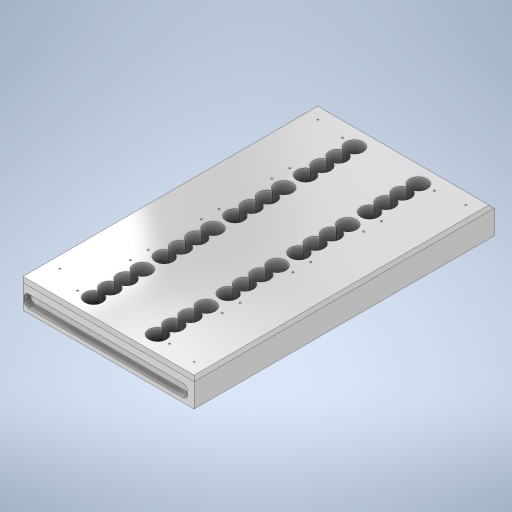
# Autodesk Inventor part: Assembly Plate
Saved by Autodesk Inventor 2023 (Build 270158000, 158)
## iProperties
Created: 2022-03-23
Part Number: Assembly Plate
Material: Generic
Document SubType Name: Modeling
Designer: Caleb
Density: 1 g/cm^3
Appearance: Aluminum - Dark
Author: Caleb
Autodesk Inventor part; units mm, degrees
ref_plane "YZ Plane" through (0, 0, 0) normal (1, 0, 0) x (0, 1, 0)
ref_plane "XZ Plane" through (0, 0, 0) normal (0, 1, 0) x (-1, 0, 0)
ref_plane "XY Plane" through (0, 0, 0) normal (0, 0, 1) x (1, 0, 0)
sketch "Sketch1" plane through (0, 0, 0) normal (0, 1, 0) x (-1, 0, 0)
  line L0 (-63.5, -107.95) -> (63.5, -107.95)
  line L1 (63.5, -107.95) -> (63.5, 107.95)
  line L2 (63.5, 107.95) -> (-63.5, 107.95)
  line L3 (-63.5, 107.95) -> (-63.5, -107.95)
  line L4 (-63.5, -107.95) -> (63.5, 107.95) construction
  line L5 (63.5, -107.95) -> (-63.5, 107.95) construction
  point P0 (0, 0)
  dimension "d0" = 127
  dimension "d1" = 215.9
  constraints: 12 end point, 2 midpoint, 2 parallel, 1 horizontal, 1 perpendicular
  measures "d0" distance of L2.end L1.end
  measures "d1" distance of L1.end L0.end
extrude "Extrusion1" add sketch "Sketch1" along normal blind 19.05
sketch "Sketch5" plane through (0, 19.05, 0) normal (0, 1, 0) x (1, 0, 0)
  line L0 (-63.5, -107.95) -> (63.5, -107.95) projected
  line L1 (63.5, 107.95) -> (-63.5, 107.95) projected
  line L2 (-63.5, 107.95) -> (-63.5, -107.95) projected
  line L3 (63.5, -107.95) -> (63.5, 107.95) projected
  point P0 (0, 0)
  point P1 (-53.15, -87.9)
  point P2 (-53.15, 97.6)
  point P3 (53.15, 97.6)
  point P4 (53.15, -97.6)
  dimension "d31" = 20.05
  dimension "d32" = 10.35
  dimension "d33" = 10.35
  dimension "d34" = 10.35
  dimension "d35" = 10.35
  dimension "d36" = 10.35
  dimension "d37" = 10.35
  dimension "d38" = 10.35
  measures "d31" distance from line of L0 point (-53.15, -87.9)
  measures "d32" distance from line of L0 point (53.15, -97.6)
  measures "d33" distance from line of L1 point (53.15, 97.6)
  measures "d34" distance from line of L1 point (-53.15, 97.6)
  measures "d35" distance from line of L2 point (-53.15, 97.6)
  measures "d36" distance from line of L3 point (53.15, 97.6)
  measures "d37" distance from line of L3 point (53.15, -97.6)
  measures "d38" distance from line of L2 point (-53.15, -87.9)
hole "Hole3" at (-53.15, 19.05, 87.9) at (-53.15, 19.05, -97.6) at (53.15, 19.05, -97.6) at (53.15, 19.05, 97.6) direction (0, -1, 0) diameter 1.0211 end through all thread size "00-96 NS" class "2B" standard "ANSI Unified Screw Threads"
sketch "Sketch6" plane through (0, 19.05, 0) normal (0, 1, 0) x (1, 0, 0)
  line L0 (-63.5, -107.95) -> (63.5, -107.95) projected
  line L1 (-63.5, 107.95) -> (-63.5, -107.95) projected
  point P0 (0, 0)
  point P1 (-25.75, -94.25)
  point P2 (-25.75, -58.15)
  point P3 (25.75, -58.15)
  point P4 (25.75, -94.25)
  point P5 (25.75, -43.45)
  point P6 (25.75, -7.35)
  point P7 (-25.75, -7.35)
  point P8 (-25.75, -43.45)
  point P9 (25.75, 7.35)
  point P10 (25.75, 43.45)
  point P11 (-25.75, 43.45)
  point P12 (-25.75, 7.35)
  point P13 (25.75, 58.15)
  point P14 (25.75, 94.25)
  point P15 (-25.75, 94.25)
  point P16 (-25.75, 58.15)
  dimension "d46" = 36.1
  dimension "d47" = 51.5
  dimension "d48" = 13.7
  dimension "d49" = 37.75
  dimension "d52" = 50.8
  constraints: 2 horizontal alignment, 2 vertical alignment, 1 vertical, 12 other
  measures "d46" distance of point (-25.75, -58.15) point (-25.75, -94.25)
  measures "d47" distance of point (25.75, -94.25) point (-25.75, -94.25)
  measures "d48" distance from line of L0 point (-25.75, -94.25)
  measures "d49" distance from line of L1 point (-25.75, -94.25)
  measures "d52" distance of point (25.75, -94.25) point (25.75, -43.45)
hole "Hole4" [suppressed]
sketch "Sketch8" plane through (63.5, 0, -107.95) normal (0, 0, -1) x (-1, 0, 0)
  line L0 (119.0625, 3.175) -> (7.9375, 3.175)
  line L1 (4.7625, 6.35) -> (4.7625, 8.89)
  line L2 (7.9375, 12.065) -> (119.0625, 12.065)
  line L3 (122.2375, 8.89) -> (122.2375, 6.35)
  line L4 (122.2375, 3.175) -> (4.7625, 12.065) construction
  line L5 (4.7625, 3.175) -> (122.2375, 12.065) construction
  line L6 (0, 0) -> (0, 19.05) projected
  line L7 (127, 0) -> (127, 19.05) projected
  line L8 (0, 0) -> (127, 0) projected
  arc A0 (7.9375, 12.065) -> (4.7625, 8.89) centre (7.9375, 8.89) ccw
  arc A1 (4.7625, 6.35) -> (7.9375, 3.175) centre (7.9375, 6.35) ccw
  arc A2 (119.0625, 3.175) -> (122.2375, 6.35) centre (119.0625, 6.35) ccw
  arc A3 (122.2375, 8.89) -> (119.0625, 12.065) centre (119.0625, 8.89) ccw
  point P0 (63.5, 0)
  point P1 (63.5, 7.62)
  point P2 (0, 15.875)
  point P3 (127, 15.875)
  dimension "d77" = 8.89
  dimension "d78" = 4.7625
  dimension "d79" = 4.7625
  dimension "d80" = 3.175
  dimension "d83" = 3.175
  constraints: 12 end point, 8 point on circle, 8 point on line, 8 tangent, 4 centre point, 3 equal radius, 2 midpoint, 2 parallel, 1 horizontal, 1 perpendicular
  measures "d77" distance of L5.start L4.end
  measures "d78" distance between parallel lines of L6 L1
  measures "d79" distance between parallel lines of L7 L3
  measures "d80" distance between parallel lines of L8 L0
  measures "d83" radius of A0
extrude "Extrusion4" cut sketch "Sketch8" against normal blind 4.7625
sketch "Sketch9" plane through (63.5, 0, 107.95) normal (0, 0, 1) x (1, 0, 0)
  line L0 (-7.9375, 3.175) -> (-119.0625, 3.175)
  line L1 (-122.2375, 6.35) -> (-122.2375, 8.89)
  line L2 (-119.0625, 12.065) -> (-7.9375, 12.065)
  line L3 (-4.7625, 8.89) -> (-4.7625, 6.35)
  line L4 (-4.7625, 3.175) -> (-122.2375, 12.065) construction
  line L5 (-122.2375, 3.175) -> (-4.7625, 12.065) construction
  arc A0 (-119.0625, 12.065) -> (-122.2375, 8.89) centre (-119.0625, 8.89) ccw
  arc A1 (-122.2375, 6.35) -> (-119.0625, 3.175) centre (-119.0625, 6.35) ccw
  arc A2 (-7.9375, 3.175) -> (-4.7625, 6.35) centre (-7.9375, 6.35) ccw
  arc A3 (-4.7625, 8.89) -> (-7.9375, 12.065) centre (-7.9375, 8.89) ccw
  line L6 (-127, 0) -> (0, 0) projected
  line L7 (-127, 0) -> (-127, 19.05) projected
  line L8 (0, 0) -> (0, 19.05) projected
  point P0 (63.5, 0)
  point P1 (-63.5, 7.62)
  point P2 (-123.825, 0)
  dimension "d84" = 8.89
  dimension "d88" = 3.175
  dimension "d89" = 3.175
  dimension "d93" = 4.7625
  dimension "d94" = 4.7625
  constraints: 12 end point, 8 point on circle, 8 point on line, 8 tangent, 4 centre point, 3 equal radius, 2 midpoint, 2 parallel, 1 horizontal, 1 perpendicular
  measures "d84" distance of L5.start L4.end
  measures "d88" radius of A0
  measures "d89" distance between parallel lines of L6 L0
  measures "d93" distance between parallel lines of L7 L1
  measures "d94" distance between parallel lines of L8 L3
extrude "Extrusion5" cut sketch "Sketch9" against normal blind 4.7625
sketch "Sketch10" plane through (0, 19.05, 0) normal (0, 1, 0) x (1, 0, 0)
  line L0 (63.5, -107.95) -> (63.5, 107.95) projected
  line L1 (-63.5, -107.95) -> (63.5, -107.95) projected
  line L2 (-63.5, 107.95) -> (-63.5, -107.95) projected
  line L3 (13.3831, -76.2) -> (-9.5437, -76.2) construction
  line L4 (0, -87.2187) -> (0, -59.9039) construction
  line L5 (13.3831, -25.4) -> (-9.5437, -25.4) construction
  line L6 (0, -36.4187) -> (0, -9.1039) construction
  line L7 (13.3831, 25.4) -> (-9.5437, 25.4) construction
  line L8 (0, 14.3813) -> (0, 41.6961) construction
  line L9 (13.3831, 76.2) -> (-9.5437, 76.2) construction
  line L10 (0, 65.1813) -> (0, 92.4961) construction
  point P0 (23, -93.7)
  point P1 (23, -82.0333)
  point P2 (-23, -93.7)
  point P3 (-23, -82.0333)
  point P4 (23, -70.3667)
  point P5 (-23, -70.3667)
  point P6 (23, -58.7)
  point P7 (-23, -58.7)
  point P8 (0, -76.2)
  point P9 (33, -95.2)
  point P10 (33, -57.2)
  point P11 (-33, -95.2)
  point P12 (-33, -57.2)
  point P13 (0, -25.4)
  point P14 (-33, -6.4)
  point P15 (-33, -44.4)
  point P16 (33, -6.4)
  point P17 (33, -44.4)
  point P18 (-23, -7.9)
  point P19 (23, -7.9)
  point P20 (-23, -19.5667)
  point P21 (23, -19.5667)
  point P22 (-23, -31.2333)
  point P23 (-23, -42.9)
  point P24 (23, -31.2333)
  point P25 (23, -42.9)
  point P26 (0, 25.4)
  point P27 (-33, 44.4)
  point P28 (-33, 6.4)
  point P29 (33, 44.4)
  point P30 (33, 6.4)
  point P31 (-23, 42.9)
  point P32 (23, 42.9)
  point P33 (-23, 31.2333)
  point P34 (23, 31.2333)
  point P35 (-23, 19.5667)
  point P36 (-23, 7.9)
  point P37 (23, 19.5667)
  point P38 (23, 7.9)
  point P39 (0, 76.2)
  point P40 (-33, 95.2)
  point P41 (-33, 57.2)
  point P42 (33, 95.2)
  point P43 (33, 57.2)
  point P44 (-23, 93.7)
  point P45 (23, 93.7)
  point P46 (-23, 82.0333)
  point P47 (23, 82.0333)
  point P48 (-23, 70.3667)
  point P49 (-23, 58.7)
  point P50 (23, 70.3667)
  point P51 (23, 58.7)
  dimension "d96" = 14.25
  dimension "d97" = 11.6667
  dimension "d127" = 11.6667
  dimension "d128" = 11.6667
  dimension "d129" = 46
  dimension "d130" = 35
  dimension "d131" = 17.5
  dimension "d132" = 23
  dimension "d133" = 33
  dimension "d134" = 19
  dimension "d135" = 38
  dimension "d136" = 33
  dimension "d146" = 50.8
  dimension "d154" = 63.5
  dimension "d155" = 127
  constraints: 16 end point, 8 point on line, 8 vertical alignment, 6 horizontal alignment, 2 perpendicular, 2 vertical, 1 horizontal, 57 other
  measures "d96" distance from line of point (23, -93.7) L1
  measures "d97" distance of point (23, -93.7) point (23, -82.033)
  measures "d127" distance of point (23, -82.033) point (23, -70.367)
  measures "d128" distance of point (23, -70.367) point (23, -58.7)
  measures "d129" distance of point (23, -93.7) point (-23, -93.7)
  measures "d130" distance of point (-23, -93.7) point (-23, -58.7)
  measures "d131" distance from line of point (-23, -58.7) L3
  measures "d132" distance from line of point (-23, -93.7) L4
  measures "d133" horizontal distance of point (33, -95.2) point (0, -76.2)
  measures "d134" vertical distance of point (33, -95.2) point (0, -76.2)
  measures "d135" distance of point (33, -57.2) point (33, -95.2)
  measures "d136" horizontal distance of point (-33, -95.2) point (0, -76.2)
  measures "d146" distance of L3.start L5.start
  measures "d154" distance from line of L0 point (0, -76.2)
  measures "d155" distance of L1.start L0.start
hole "Hole5" at (23, 19.05, 93.7) at (23, 19.05, 82.0333) at (-23, 19.05, 93.7) at (-23, 19.05, 82.0333) at (23, 19.05, 70.3667) at (23, 19.05, 58.7) at (-23, 19.05, 58.7) at (-23, 19.05, 70.3667) at (-23, 19.05, -58.7) at (-23, 19.05, -70.3667) at (-23, 19.05, -82.0333) at (-23, 19.05, -93.7) at (-23, 19.05, -7.9) at (-23, 19.05, -19.5667) at (-23, 19.05, -31.2333) at (-23, 19.05, -42.9) at (-23, 19.05, 42.9) at (-23, 19.05, 31.2333) at (-23, 19.05, 19.5667) at (-23, 19.05, 7.9) at (23, 19.05, -58.7) at (23, 19.05, -70.3667) at (23, 19.05, -82.0333) at (23, 19.05, -93.7) at (23, 19.05, -7.9) at (23, 19.05, -19.5667) at (23, 19.05, -31.2333) at (23, 19.05, -42.9) at (23, 19.05, 42.9) at (23, 19.05, 31.2333) at (23, 19.05, 19.5667) at (23, 19.05, 7.9) direction (0, -1, 0) diameter 3.9624 end through all counterbore diameter 12.7 counterbore depth 15.494 thread size "10-32 UNF" class "2B" standard "ANSI Unified Screw Threads"
chamfer "Chamfer3" distance 2 angle 45 4 edges at (63.5, 19.05, 0) (0, 19.05, 107.95) (-63.5, 19.05, 0) (0, 19.05, -107.95)
sketch "Sketch11" plane through (0, 0, 0) normal (0, -1, 0) x (1, 0, 0)
  line L0 (12, -91.95) -> (-12, -91.95)
  line L1 (-14, -89.95) -> (-14, 89.95)
  line L2 (-12, 91.95) -> (12, 91.95)
  line L3 (14, 89.95) -> (14, -89.95)
  line L4 (-34, -91.95) -> (-43.5, -91.95)
  line L5 (-45.5, -89.95) -> (-45.5, 89.95)
  line L6 (-43.5, 91.95) -> (-34, 91.95)
  line L7 (-32, 89.95) -> (-32, -89.95)
  circle A0 centre (53.15, 97.6) radius 0.5105 projected
  line L8 (34, -91.95) -> (43.5, -91.95)
  line L9 (45.5, -89.95) -> (45.5, 89.95)
  line L10 (43.5, 91.95) -> (34, 91.95)
  line L11 (32, 89.95) -> (32, -89.95)
  line L12 (-63.5, 107.95) -> (63.5, 107.95) projected
  line L13 (-63.5, -107.95) -> (-63.5, 107.95) projected
  line L14 (63.5, 107.95) -> (63.5, -107.95) projected
  circle A1 centre (23, 93.7) radius 1.9812 projected
  circle A2 centre (-23, 93.7) radius 1.9812 projected
  line L15 (63.5, -107.95) -> (-63.5, -107.95) projected
  arc A3 (-43.5, 91.95) -> (-45.5, 89.95) centre (-43.5, 89.95) ccw
  arc A4 (-32, 89.95) -> (-34, 91.95) centre (-34, 89.95) ccw
  arc A5 (-45.5, -89.95) -> (-43.5, -91.95) centre (-43.5, -89.95) ccw
  arc A6 (-34, -91.95) -> (-32, -89.95) centre (-34, -89.95) ccw
  arc A7 (-14, -89.95) -> (-12, -91.95) centre (-12, -89.95) ccw
  arc A8 (12, -91.95) -> (14, -89.95) centre (12, -89.95) ccw
  arc A9 (-12, 91.95) -> (-14, 89.95) centre (-12, 89.95) ccw
  arc A10 (14, 89.95) -> (12, 91.95) centre (12, 89.95) ccw
  arc A11 (34, 91.95) -> (32, 89.95) centre (34, 89.95) ccw
  arc A12 (45.5, 89.95) -> (43.5, 91.95) centre (43.5, 89.95) ccw
  arc A13 (32, -89.95) -> (34, -91.95) centre (34, -89.95) ccw
  arc A14 (43.5, -91.95) -> (45.5, -89.95) centre (43.5, -89.95) ccw
  point P0 (0, 0)
  point P1 (-32, -91.95)
  point P2 (-45.5, 91.95)
  point P3 (32, -91.95)
  point P4 (45.5, 91.95)
  point P5 (53.1436, 97.0895)
  point P6 (52.6395, 97.5936)
  dimension "d116" = 16
  dimension "d117" = 18
  dimension "d118" = 18
  dimension "d119" = 9
  dimension "d120" = 9
  dimension "d121" = 9
  dimension "d122" = 9
  dimension "d123" = 16
  dimension "d124" = 2
  constraints: 24 end point, 24 point on circle, 24 tangent, 12 centre point, 12 point on line, 11 equal radius, 6 parallel, 3 horizontal, 3 perpendicular
  measures "d116" distance between parallel lines of L12 L6
  measures "d117" distance between parallel lines of L13 L5
  measures "d118" distance between parallel lines of L14 L9
  measures "d119" distance from line of A1.centre L11
  measures "d120" distance from line of A1.centre L3
  measures "d121" distance from line of L1 A2.centre
  measures "d122" distance from line of L7 A2.centre
  measures "d123" distance between parallel lines of L15 L4
  measures "d124" radius of A3
extrude "Extrusion6" cut sketch "Sketch11" against normal blind 12.7 contours L0 A7 L1 A9 L2 A10 L3 A8 | L4 A5 L5 A3 L6 A4 L7 A6 | A13 L11 A11 L10 A12 L9 A14 L8
hole "Hole6" at (-33, 19.05, 95.2) at (-33, 19.05, 57.2) at (33, 19.05, 57.2) at (33, 19.05, 95.2) at (33, 19.05, -57.2) at (33, 19.05, -95.2) at (33, 19.05, -6.4) at (33, 19.05, -44.4) at (33, 19.05, 44.4) at (33, 19.05, 6.4) at (-33, 19.05, -57.2) at (-33, 19.05, -95.2) at (-33, 19.05, -6.4) at (-33, 19.05, -44.4) at (-33, 19.05, 44.4) at (-33, 19.05, 6.4) direction (0, -1, 0) diameter 1.1811 end through all thread size "0-80 UNF" class "2B" standard "ANSI Unified Screw Threads"
chamfer "Chamfer4" distance 4 angle 45 1 edges at (-63.5, 8.525, 107.95)
equation "\"d79\" = d78"
equation "\"d128\" = d97"
equation "\"d131\" = 0.5 * d130"
equation "\"d132\" = 0.5 * d129"
equation "\"d135\" = 2 * d134"
equation "\"d136\" = d133"
equation "\"d154\" = 0.5 * d155"
body "Solid1"
